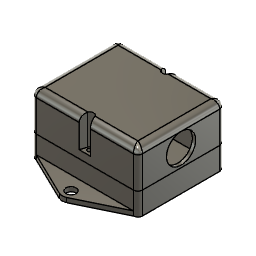
Case sensor ultrasonico v0 (Autodesk Fusion 360 design; units mm, degrees)
Autodesk Fusion 360 part; units mm, degrees
sketch "Sketch1" plane through (0, 0, 0) normal (0, 1, 0) x (1, 0, 0)
  line L0 (0, 0) -> (41.3, 0)
  line L1 (41.3, 0) -> (41.3, 28.5)
  line L2 (41.3, 28.5) -> (0, 28.5)
  line L3 (0, 28.5) -> (0, 0)
  line L4 (20.65, 28.5) -> (20.65, 0) construction
  line L5 (0, 14.25) -> (41.3, 14.25) construction
  circle A0 centre (2.65, 26.25) radius 1.15
  line L6 (-1, -5) -> (42.3, -5)
  line L7 (44.3, -3) -> (44.3, 31.5)
  line L8 (42.3, 33.5) -> (-1, 33.5)
  line L9 (-3, 31.5) -> (-3, -3)
  arc A1 (-1, 33.5) -> (-3, 31.5) centre (-1, 31.5) ccw
  arc A2 (-3, -3) -> (-1, -5) centre (-1, -3) ccw
  arc A3 (42.3, -5) -> (44.3, -3) centre (42.3, -3) ccw
  arc A4 (44.3, 31.5) -> (42.3, 33.5) centre (42.3, 31.5) ccw
  circle A5 centre (2.65, 26.25) radius 2.75
  circle A6 centre (38.65, 26.25) radius 2.75
  circle A7 centre (38.65, 26.25) radius 1.15
  circle A8 centre (38.65, 2.25) radius 1.15
  circle A9 centre (38.65, 2.25) radius 2.75
  circle A10 centre (2.65, 2.25) radius 1.15
  circle A11 centre (2.65, 2.25) radius 2.75
  circle A12 centre (20.65, 31.2469) radius 0.875
  circle A13 centre (20.65, 31.2469) radius 1
  circle A14 centre (20.65, -2.7469) radius 0.875
  circle A15 centre (20.65, -2.7469) radius 1
  dimension "d1" = 41.3
  dimension "d2" = 28.5
  dimension "d3" = 2.3
  dimension "d4" = 12
  dimension "d5" = 18
  dimension "d7" = 2
  dimension "d8" = 5.5
  dimension "d29" = 1.75
  dimension "d30" = 2
  constraint horizontal L0
  constraint vertical L1
  constraint horizontal L2
  constraint vertical L3
  constraint coincident L0.start L3.end
  constraint midpoint L2 L4.start
  constraint midpoint L0 L4.end
  constraint midpoint L3 L5.start
  constraint midpoint L1 L5.end
  constraint tangent L8 A1
  constraint tangent L9 A1
  constraint tangent L6 A2
  constraint tangent L9 A2
  constraint equal A1 A2
  constraint tangent L6 A3
  constraint tangent L7 A3
  constraint equal A1 A3
  constraint tangent L7 A4
  constraint tangent L8 A4
  constraint equal A1 A4
  constraint concentric A0 A5
  constraint symmetric L4 A0 A7
  constraint symmetric L4 A5 A6
  constraint symmetric L5 A0 A10
  constraint symmetric L5 A5 A11
  constraint symmetric L5 A6 A9
  constraint symmetric L5 A7 A8
  constraint symmetric L5 A12 A14
  constraint symmetric L5 A13 A15
  measures "d1" distance of L0.start L0.end
  measures "d2" distance of L0.start L2.end
  measures "d3" diameter of A0
  measures "d4" distance of L5 A0.centre
  measures "d5" distance of L4 A0.centre
  measures "d7" radius of A1
  measures "d8" diameter of A5
  measures "d29" diameter of A12
  measures "d30" diameter of A13
extrude "Extrude1" add sketch "Sketch1" along normal blind 27 contours L0 L3 A11 | L0 L3 A11 | L0 A11 | L3 A11 | L0 L1 L2 L3 A5 A6 A9 A11 | L0 L1 A9 | L0 A9 | L3 A5 | L2 L3 A5 | L0 L1 A9 | L1 A9 | L2 L3 A5 | L1 L2 A6 | L1 A6 | L2 A5 | L1 L2 A6 | L2 A6 | A0 | L6 L7 L8 L9 A1 A2 A3 A4 | A7 | A8 | A10 | A12 | A13 | A14 | A15 makes body 1
sketch "Sketch2" plane through (44.3, 0, 0) normal (1, 0, 0) x (0, 0, -1)
  line L0 (-3, 0) -> (31.5, 0)
  line L1 (31.5, 0) -> (31.5, 27)
  line L2 (31.5, 27) -> (-3, 27)
  line L3 (-3, 27) -> (-3, 0)
  line L4 (14.25, 27) -> (14.25, 0) construction
  circle A0 centre (14.25, 17.5) radius 8
  circle A1 centre (14.25, 17.5) radius 6.5
  dimension "d11" = 16
  dimension "d12" = 13
  dimension "d13" = 9.5
  constraint midpoint L2 L4.start
  constraint midpoint L0 L4.end
  constraint coincident L4 A0.centre
  constraint concentric A0 A1
  measures "d11" diameter of A0
  measures "d12" diameter of A1
  measures "d13" distance of L4.start A0.centre
ref_plane "WorkPlane3" through (0, 10, 0) normal (0, 1, 0) x (0, 0, 1)
split "Split2" by plane through (0, 10, 0) normal (0, 1, 0) bodies 1 makes body 2 at (27.8667, 27, -7.8333)
shell "Shell3" thickness 1.5 removed faces 1 at (13.4333, 10, -7.8333) on bodies 1
shell "Shell4" thickness 1.5 removed faces 1 at (13.4333, 10, -7.8333) on bodies 2
sketch "Sketch5" plane through (0, 0, 0) normal (0, 1, 0) x (1, 0, 0)
  line L0 (18.4936, 30.6046) -> (17.6312, 33.5)
  line L1 (20.65, 31.2469) -> (20.65, -2.7469) construction
  line L2 (22.8064, 30.6046) -> (23.6688, 33.5)
  line L3 (17.6312, 33.5) -> (23.6688, 33.5)
  arc A0 (18.4936, 30.6046) -> (22.8064, 30.6046) centre (20.65, 31.2469) ccw
  line L4 (22.3272, 30.7474) -> (23.1471, 33.5)
  arc A1 (18.9728, 30.7474) -> (22.3272, 30.7474) centre (20.65, 31.2469) ccw
  line L5 (18.9728, 30.7474) -> (18.1529, 33.5)
  line L6 (0, 14.25) -> (41.3, 14.25)
  line L7 (22.8064, -2.1046) -> (23.6688, -5)
  arc A2 (22.8064, -2.1046) -> (18.4936, -2.1046) centre (20.65, -2.7469) ccw
  line L8 (18.4936, -2.1046) -> (17.6312, -5)
  line L9 (22.3272, -2.2474) -> (23.1471, -5)
  arc A3 (22.3272, -2.2474) -> (18.9728, -2.2474) centre (20.65, -2.7469) ccw
  line L10 (18.9728, -2.2474) -> (18.1529, -5)
  line L11 (17.6312, -5) -> (23.6688, -5)
  point P0 (20.65, 31.2469)
  point P1 (17.6312, 33.5)
  point P2 (20.65, -2.7469)
  dimension "d49" = 4.5
  dimension "d50" = -0.5
  constraint coincident P0 L1.start
  constraint coincident P1 L0.end
  constraint coincident P2 L1.end
  constraint symmetric L0.start L1 L2.start
  constraint symmetric P1 L1 L2.end
  constraint coincident L3 L4.end
  constraint coincident L3 L5.end
  constraint symmetric L0.start L6 A2.end
  constraint symmetric P1 L6 L8.end
  constraint symmetric L2.start L6 L7.start
  constraint symmetric L2.end L6 L7.end
  constraint symmetric A0 L6 A2
  constraint symmetric L4.start L6 L9.start
  constraint symmetric L4.end L6 L9.end
  constraint symmetric A1.start L6 A3.end
  constraint symmetric A1 L6 A3
  constraint symmetric L5.end L6 L10.end
  measures "d49" diameter of A0
extrude "Extrude9" add sketch "Sketch5" along normal blind 10 bodies 1
extrude "Extrude10" add sketch "Sketch1" sketch "Sketch5" along normal blind 17 from surface at 10 contours A12 | A13 of sketch 2 bodies 2
fillet "Fillet3" radius 3 8 edges at (44.3, 27, -14.25) (43.7142, 27, -32.9142) (20.65, 27, -33.5) (-2.4142, 27, -32.9142) (-3, 27, -14.25) (-2.4142, 27, 4.4142) (20.65, 27, 5) (43.7142, 27, 4.4142) on bodies 2
extrude "Extrude11" cut sketch "Sketch5" along normal blind 21 from surface at 13.5 contours L3 L4 A1 L5 | L9 A3 L10 L11 bodies 2
extrude "Extrude12" cut sketch "Sketch1" along normal blind 18.5 contours A12 | A13 | A14 | A15 bodies 2
extrude "Extrude13" cut sketch "Sketch1" along normal blind 11 from surface at 5 contours A12 | A14 bodies 1
extrude "Extrude14" cut sketch "Sketch2" against normal blind 8 contours A1 bodies 2
sketch "Sketch6" plane through (0, 0, 0) normal (0, 1, 0) x (1, 0, 0)
  circle A0 centre (20.65, 39.6338) radius 2.25
  line L0 (19.1487, 43.2771) -> (-1, 33.5)
  line L1 (20.65, 31.2469) -> (20.65, -2.7469)
  line L2 (22.1513, 43.2771) -> (42.3, 33.5)
  arc A1 (22.1513, 43.2771) -> (19.1487, 43.2771) centre (20.65, 39.6338) ccw
  line L3 (-1, 33.5) -> (42.3, 33.5)
  line L4 (0, 14.25) -> (41.3, 14.25)
  circle A2 centre (20.65, -11.1338) radius 2.25
  line L5 (22.1513, -14.7771) -> (42.3, -5)
  line L6 (-1, -5) -> (42.3, -5)
  line L7 (19.1487, -14.7771) -> (-1, -5)
  arc A3 (19.1487, -14.7771) -> (22.1513, -14.7771) centre (20.65, -11.1338) ccw
  circle A4 centre (2.65, 26.25) radius 0.9658
  line L8 (20.65, 28.5) -> (20.65, 0)
  circle A5 centre (38.65, 26.25) radius 0.9658
  circle A6 centre (38.65, 2.25) radius 0.9658
  circle A7 centre (2.65, 2.25) radius 0.9658
  point P0 (-1, 33.5)
  point P1 (20.65, 28.5)
  point P2 (20.65, 31.2469)
  point P3 (2.65, 26.25)
  dimension "d71" = 4.5
  dimension "d72" = 3.9405
  dimension "d73" = 8.3869
  constraint concentric A0 A1
  constraint coincident P0 L0.end
  constraint vertical A0.centre P1
  constraint symmetric L0.start L1 L2.start
  constraint symmetric P0 L1 L2.end
  constraint symmetric A0 L4 A2
  constraint symmetric L0.start L4 L7.start
  constraint symmetric P0 L4 L6.start
  constraint symmetric L2.start L4 L5.start
  constraint symmetric L2.end L4 L5.end
  constraint symmetric A1 L4 A3
  constraint coincident P3 A4.centre
  constraint symmetric A4 L8 A5
  constraint symmetric L4 A4 A7
  constraint symmetric L4 A5 A6
  measures "d71" diameter of A0
  measures "d72" radius of A1
  measures "d73" distance of A0.centre P2
extrude "Extrude16" add sketch "Sketch6" along normal blind 2 contours L0 L2 A1 L3 | L5 L6 L7 A3 bodies 1
extrude "Extrude19" add sketch "Sketch1" sketch "Sketch6" along normal blind 5 contours L0 L3 A11 | L0 A11 | L3 A11 | L0 L1 A9 | L0 A9 | L1 A9 | L1 L2 A6 | L1 A6 | L2 A6 | A7 | A8 | A10 picked at (2.6786, 0.3677) picked at (38.6214, 0.3677) picked at (38.6214, 28.1323) of sketch 2 contours A7 bodies 1
extrude "Extrude20" cut sketch "Sketch6" along normal blind 9 from surface at 2 contours A4 | A5 | A6 | A7 bodies 1
equation "d4 = ( 24 / 2 ) * 1 mm"
equation "d5 = ( 36 / 2 ) * 1 mm"
